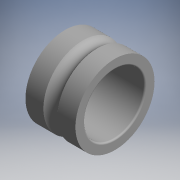
# Autodesk Inventor part: WA673SA Inner ring
Saved by Autodesk Inventor 2017.3 (Build 213256000, 256)
## iProperties
Part Number: WA673SA Inner ring
Material: Generic
Catalog Web Link: www.cadenas.de
Description: Six types ir-Metric system sizes
Vendor: NTN
Document SubType Name: Modeling
Designer: partserver
Manufacturer: NTN
Mass: 0.0120659 g
Surface Area: 0.652944 cm^2
Volume: 0.0120659 cm^3
Density: 1 g/cm^3
Appearance: PSOLRGB-192-192-192
Category: PARTsolutions
Company: NTN
Title: WA673SA Inner ring
Author: Cadenas PARTsolutions
Comments: Metric system sizes
PSOL_IDENT_0: {$CADENAS_DATA\23d-libs\ntn\ball_roller_bearings\miniature_extra_small_bb\metric_system_sizes\mss_ir
PSOL_IDENT_1: .prj},185 {VTYP=3D},{NB=WA673SA Inner ring},{LINA=WA673SA Inner ring},{NN=Six types ir},{DATE=21.12.
PSOL_IDENT_2: 2021 04:23:04},{GEOMDATE=06.03.2020 10:06:06},{VERSION=},{LINEID=11430},{WBVAR=},{WBNUMERIC=}  {NB=W
PSOL_IDENT_3: A673SA Inner ring},{LINA=WA673SA Inner ring},{KT=DUMMY},{IDNR=},{SD=3.0},{D=6},{B=2.0},{R=0.08},{ORD
PSOL_IDENT_4: ER=WA673SA},{CR=242},{COR=94},{CRF=25},{CORF=9,5},{LSG=60 000},{LSO=71 000},{MASS=0.20},{D1=7.2},{D2=
PSOL_IDENT_5: 7.2},{C1=0.6},{C2=0.6},{ORDER1=673},{WSS=WA673SA},{WDS=SSA},{UTWF=FL673},{FORSS=FLWA673SA},{FORDS=SS
PSOL_IDENT_6: A},{DA1=3,6},{DA2=4,1},{DA=5,4},{RAS=0,08},{MASS1=0.26},{B1=2.5},{VERS=2},{X=1.5},{N=9},{O=14.13},{R
PSOL_IDENT_7: B=0.444}
NB: WA673SA Inner ring
NN: Six types ir
NT: Metric system sizes
NBSYN: $ORDER. Inner ring
LINA: WA673SA Inner ring
CATALOG: NTN Corporation
SD: 3
D: 6
B: 2
R: 0.08
CR: 242
COR: 94
CRF: 25
CORF: 9,5
LSG: 60 000
LSO: 71 000
MASS: 0.2
D1: 7.2
D2: 7.2
C1: 0.6
C2: 0.6
ORDER1: 673
WSS: WA673SA
WDS: SSA
UTWF: FL673
FORSS: FLWA673SA
FORDS: SSA
DA1: 3,6
DA2: 4,1
DA: 5,4
RAS: 0,08
MASS1: 0.26
B1: 2.5
VERS: 2
SUPPLIER: NTN
ARTICLENO: WA673SA Inner ring
BOMINFO: WA673SA Inner ring
CREATOR: CADENAS GmbH
Autodesk Inventor part; units mm, degrees
sketch "Sketch_2" plane through (0, 0, 0) normal (0, 0, 1) x (1, 0, 0)
  line L0 (2.5, 0) -> (0, 0)
  arc A0 (0, 1.58) -> (0.08, 1.5) centre (0.08, 1.58) ccw
  line L1 (0.08, 1.5) -> (2.42, 1.5)
  arc A1 (2.42, 1.5) -> (2.5, 1.58) centre (2.42, 1.58) ccw
  line L2 (2.5, 1.58) -> (2.5, 1.98)
  line L3 (2.5, 1.98) -> (1.6025, 1.98)
  arc A2 (0.8975, 1.98) -> (1.6025, 1.98) centre (1.25, 2.25) ccw
  line L4 (0.8975, 1.98) -> (0, 1.98)
  line L5 (0, 1.98) -> (0, 1.58)
  constraints: 12 end point, 6 point on circle, 3 centre point
revolve "Revolution1" add sketch "Sketch_2" angle 360 about axis through (2.5, 0, 0) along (1, 0, 0)
ref_plane "mss_ir_XY" through (0, 0, 0) normal (1, 0, 0) x (0, 0, -1)
ref_plane "mss_ir_YZ" through (0, 0, 0) normal (0, 0, -1) x (0, 1, 0)
ref_plane "mss_ir_ZX" through (0, 0, 0) normal (0, 1, 0) x (1, 0, 0)
body "Solid1"
